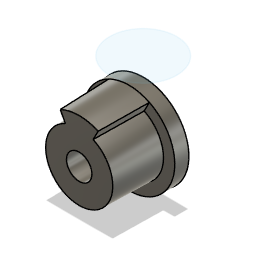
西昊C300头部支撑固定桩 (Autodesk Fusion 360 design; units mm, degrees)
Autodesk Fusion 360 part; units mm, degrees
sketch "草图1" plane through (0, 0, 0) normal (0, 1, 0) x (1, 0, 0)
  circle A0 centre (0, 0) radius 10.35
  dimension "d1" = 20.7
  constraint coincident A0.centre origin
  measures "d1" diameter of A0
extrude "拉伸1" add sketch "草图1" along normal blind 14.5 contours A0 picked at (-1.590097, 1.26806)
sketch "草图2" plane through (0, 14.5, 0) normal (0, 1, 0) x (-1, 0, 0)
  circle A0 centre (0, 0) radius 10.35
  circle A1 centre (0, 0) radius 7.6
  dimension "d4" = 15.2
  constraint coincident A0.centre A1.centre
  measures "d4" diameter of A1
extrude "拉伸2" cut sketch "草图2" against normal blind 11.3 draft -1 contours A0 picked at (9.3948, -0.514196)
sketch "草图3" plane through (0, 14.5, 0) normal (0, 1, 0) x (-1, 0, 0)
  circle A0 centre (0, 0) radius 7.6
  circle A1 centre (0, 0) radius 11.176414
  circle A2 centre (0, 0) radius 9.823441
  constraint coincident A0.centre A1.centre
  constraint concentric A1 A2
extrude "拉伸3" cut sketch "草图3" against normal blind 11.3 contours A1 picked at (10.683813, -0.555253)
sketch "草图6" plane through (0, 3.2, 0) normal (0, 1, 0) x (-1, 0, 0)
  circle A0 centre (0, 0) radius 10.35
  circle A1 centre (0, 0) radius 7.797242
  circle A2 centre (0, 0) radius 10.35
  line L0 (5.18, -3.9) -> (-5.15, -3.9)
  line L1 (-5.15, -3.9) -> (-5.15, -8.97775)
  line L2 (-5.15, -8.97775) -> (5.18, -8.97775)
  line L3 (5.18, -8.97775) -> (5.18, -3.9)
  dimension "d16" = 20.7
  dimension "d18" = 5.15
  dimension "d20" = 10.33
  constraint concentric A0 A2
  constraint horizontal L0
  constraint vertical L1
  constraint horizontal L2
  constraint vertical L3
  measures "d16" diameter of A2
  measures "d18" distance of A0.centre L1
  measures "d20" distance of L1 L3
extrude "拉伸5" add sketch "草图6" along normal blind 11.3 draft -1.5 contours A0 A2 L2 | A0 A1 A2 L1 L2 L3 picked at (1.254031, -9.199184) picked at (0.006674, -8.584239)
sketch "草图7" plane through (0, 14.5, 0) normal (0, 1, 0) x (-1, 0, 0)
  circle A0 centre (0, 0) radius 7.6
sketch "草图8" plane through (0, 14.5, 0) normal (0, 1, 0) x (-1, 0, 0)
sketch "草图9" plane through (0, 14.5, 0) normal (0, 1, 0) x (-1, 0, 0)
sketch "草图10" plane through (0, 14.5, 0) normal (0, 1, 0) x (-1, 0, 0)
  line L0 (-4.854099, -6.475854) -> (-4.854099, -8.804694)
  arc A0 (-4.854099, -8.804694) -> (4.884099, -8.788088) centre (0, 0) ccw
  line L1 (4.884099, -8.788088) -> (4.884099, -6.453258)
  arc A1 (-4.854099, -6.475854) -> (4.884099, -6.453258) centre (0, 0) ccw
  line L2 (4.884099, -6.453258) -> (-4.854099, -6.475854)
  line L3 (0, 0) -> (4.884099, 0)
  line L4 (4.884099, 0) -> (4.884099, -6.453258)
  line L5 (4.884099, -6.453258) -> (0, -6.453258)
  line L6 (0, -6.453258) -> (0, 0)
  line L7 (0, 0) -> (-4.854099, 0)
  line L8 (-4.854099, 0) -> (-4.854099, -6.475854)
  line L9 (-4.854099, -6.475854) -> (0, -6.475854)
  line L10 (0, -6.475854) -> (0, 0)
  constraint horizontal L3
  constraint vertical L4
  constraint horizontal L5
  constraint vertical L6
  constraint coincident A0.centre A1.centre
  constraint horizontal L7
  constraint vertical L8
  constraint horizontal L9
  constraint vertical L10
extrude "拉伸6" add sketch "草图10" against normal blind 11.3 draft 1.5 contours A1 L2 L9 L10 | L2 L6 L7 L8 L10 | L3 L4 L5 L6 L10 picked at (0.012487, -7.540159) picked at (-3.236066, -4.309704) picked at (1.628033, -4.302172)
sketch "草图11" plane through (0, 14.5, 0) normal (0, 1, 0) x (-1, 0, 0)
sketch "草图12" plane through (0, 14.5, 0) normal (0, 1, 0) x (-1, 0, 0)
  line L0 (-4.854099, -6.475854) -> (-4.854099, -8.804694)
  arc A0 (-4.854099, -8.804694) -> (4.884099, -8.788088) centre (0, 0) ccw
  line L1 (4.884099, -8.788088) -> (4.884099, -6.453258)
  line L2 (4.884099, -6.453258) -> (4.011148, -6.455284)
  arc A1 (4.011148, -6.455284) -> (4.014406, -6.453258) centre (0, 0) ccw
  line L3 (4.014406, -6.453258) -> (4.884099, -6.453258)
  line L4 (4.884099, -6.453258) -> (4.884099, -5.822849)
  arc A2 (4.884099, -5.822849) -> (-4.854099, -5.847882) centre (0, 0) ccw
  line L5 (-4.854099, -5.847882) -> (-4.854099, -6.475854)
  line L6 (-4.854099, -6.475854) -> (-3.981148, -6.473829)
  arc A3 (-3.981148, -6.473829) -> (-3.977853, -6.475854) centre (0, 0) ccw
  line L7 (-3.977853, -6.475854) -> (-4.854099, -6.475854)
  line L8 (-4.854099, -5.847882) -> (-4.854099, -8.804694)
  line L9 (4.884099, -8.788088) -> (4.884099, -5.822849)
  line L10 (6.095858, -5.822849) -> (6.095858, -8.804694)
  line L11 (6.095858, -8.804694) -> (4.884099, -8.788088)
  line L12 (6.095858, -5.822849) -> (4.884099, -5.822849)
  line L13 (-4.854099, -8.804694) -> (-6, -8.804694)
  line L14 (-6, -8.804694) -> (-6, -5.822849)
  line L15 (-6, -5.822849) -> (-4.854099, -5.847882)
  constraint parallel L4 L10
  constraint perpendicular L4 L12
  constraint perpendicular L8 L13
  constraint perpendicular L13 L14
extrude "拉伸7" cut sketch "草图12" against normal blind 11.3 draft -1.5 contours L0 L5 L8 L13 L14 L15 | L1 L4 L9 L10 L11 L12 picked at (-5.618033, -7.034466) picked at (5.691938, -7.026934)
sketch "草图13" plane through (0, 0, 0) normal (0, -1, 0) x (1, 0, 0)
  circle A0 centre (0, 0) radius 10.35
  circle A1 centre (0, 0) radius 3.1
  dimension "d28" = 6.2
  constraint concentric A0 A1
  measures "d28" diameter of A1
extrude "拉伸8" cut sketch "草图13" against normal blind 14.5 draft -0.85 contours A1 picked at (-0.459877, 1.40569)
sketch "草图15" plane through (0, 3.2, 0) normal (0, 1, 0) x (-1, 0, 0)
  line L0 (5.18, -5.827914) -> (5.18, -8.960474)
  arc A0 (5.18, -8.960474) -> (-5.15, -8.97775) centre (0, 0) ccw
  line L1 (-5.15, -8.97775) -> (-5.15, -5.854442)
  arc A1 (5.18, -5.827914) -> (-5.15, -5.854442) centre (0, 0) ccw
  line L2 (5.18, -5.827914) -> (-0.020023, -5.827914)
  line L3 (-0.020023, -5.827914) -> (-0.020023, -10.347219)
  line L4 (-0.020023, -10.347219) -> (5.18, -10.347219)
  line L5 (5.18, -10.347219) -> (5.18, -5.827914)
  line L6 (-5.15, -5.854442) -> (-0.020023, -5.854442)
  line L7 (-0.020023, -5.854442) -> (-0.020023, -10.347219)
  line L8 (-0.020023, -10.347219) -> (-5.15, -10.347219)
  line L9 (-5.15, -10.347219) -> (-5.15, -5.854442)
  line L10 (-0.020023, -5.827914) -> (2.779977, -5.827914)
  line L11 (2.779977, -5.827914) -> (2.779977, -10.347219)
  line L12 (2.779977, -10.347219) -> (-0.020023, -10.347219)
  line L13 (-0.020023, -10.347219) -> (-0.020023, -5.827914)
  line L14 (-0.020023, -5.854442) -> (-2.820023, -5.854442)
  line L15 (-2.820023, -5.854442) -> (-2.820023, -10.347219)
  line L16 (-2.820023, -10.347219) -> (-0.020023, -10.347219)
  line L17 (-0.020023, -10.347219) -> (-0.020023, -5.854442)
  circle A2 centre (0, 0) radius 7.797242
  line L18 (5.18, -10.347219) -> (2.779977, -5.827914)
  line L19 (-5.15, -10.347219) -> (-2.820023, -5.854442)
  dimension "d33" = 2.8
  dimension "d34" = 2.8
  constraint horizontal L2
  constraint vertical L3
  constraint horizontal L4
  constraint vertical L5
  constraint horizontal L6
  constraint vertical L7
  constraint horizontal L8
  constraint vertical L9
  constraint horizontal L10
  constraint vertical L11
  constraint horizontal L12
  constraint vertical L13
  constraint horizontal L14
  constraint vertical L15
  constraint horizontal L16
  constraint vertical L17
  constraint concentric A0 A2
extrude "拉伸9" cut sketch "草图15" along normal blind 11.3 draft 1 contours L0 L5 A2 L18 | L1 L9 A2 L19 picked at (4.589689, -8.7734) picked at (-4.572759, -8.777664)
move_body "移动1" bodies 1 to x (1, 0, 0) y (0, 0, 1) z (0, -1, 0) at (0, 0, 0)
sketch "草图14" plane through (0, 14.5, 0) normal (0, 1, 0) x (-1, 0, 0)
  circle A0 centre (0, 0) radius 2.884872
  line L0 (-4.854099, -6.475854) -> (-4.854099, -8.804694)
  arc A1 (-4.854099, -8.804694) -> (4.884099, -8.788088) centre (0, 0) ccw
  line L1 (4.884099, -8.788088) -> (4.884099, -6.453258)
  line L2 (4.884099, -6.453258) -> (4.011148, -6.455284)
  arc A2 (4.011148, -6.455284) -> (4.014406, -6.453258) centre (0, 0) ccw
  line L3 (4.014406, -6.453258) -> (4.884099, -6.453258)
  line L4 (4.884099, -6.453258) -> (4.884099, -5.822849)
  arc A3 (4.884099, -5.822849) -> (-4.854099, -5.847882) centre (0, 0) ccw
  line L5 (-4.854099, -5.847882) -> (-4.854099, -6.475854)
  line L6 (-4.854099, -6.475854) -> (-3.981148, -6.473829)
  arc A4 (-3.981148, -6.473829) -> (-3.977853, -6.475854) centre (0, 0) ccw
  line L7 (-3.977853, -6.475854) -> (-4.854099, -6.475854)
  line L8 (-4.854099, -5.847882) -> (0.017145, -5.847882)
  line L9 (0.017145, -5.847882) -> (0.017145, -10.054084)
  line L10 (0.017145, -10.054084) -> (-4.854099, -10.054084)
  line L11 (-4.854099, -10.054084) -> (-4.854099, -5.847882)
  line L12 (4.884099, -5.822849) -> (0.017145, -5.822849)
  line L13 (0.017145, -5.822849) -> (0.017145, -10.054084)
  line L14 (0.017145, -10.054084) -> (4.884099, -10.054084)
  line L15 (4.884099, -10.054084) -> (4.884099, -5.822849)
  line L16 (0.017145, -10.054084) -> (2.817145, -10.054084)
  line L17 (2.817145, -10.054084) -> (2.817145, -5.822849)
  line L18 (2.817145, -5.822849) -> (0.017145, -5.822849)
  line L19 (0.017145, -5.822849) -> (0.017145, -10.054084)
  line L20 (0.017145, -10.054084) -> (-2.782855, -10.054084)
  line L21 (-2.782855, -10.054084) -> (-2.782855, -5.847882)
  line L22 (-2.782855, -5.847882) -> (0.017145, -5.847882)
  line L23 (0.017145, -5.847882) -> (0.017145, -10.054084)
  circle A5 centre (0, 0) radius 7.6
  line L24 (4.884099, -8.788088) -> (2.817145, -5.822849)
  line L25 (-4.854099, -8.804694) -> (-2.782855, -5.847882)
  dimension "d31" = 2.8
  dimension "d32" = 2.8
  constraint horizontal L8
  constraint vertical L9
  constraint horizontal L10
  constraint vertical L11
  constraint horizontal L12
  constraint vertical L13
  constraint horizontal L14
  constraint vertical L15
  constraint horizontal L16
  constraint vertical L17
  constraint horizontal L18
  constraint vertical L19
  constraint horizontal L20
  constraint vertical L21
  constraint horizontal L22
  constraint vertical L23
  constraint concentric A0 A5
sketch "草图4" plane through (0, 14.5, 0) normal (0, 1, 0) x (-1, 0, 0)
  circle A0 centre (0, 0) radius 7.6
  line L0 (7.6, -10.35) -> (-7.6, -10.35)
  line L1 (-7.6, -10.35) -> (-7.6, -7.6)
  line L2 (-7.6, -7.6) -> (7.6, -7.6)
  line L3 (7.6, -7.6) -> (7.6, -10.35)
  circle A1 centre (0, -10.35) radius 7.6
  circle A2 centre (0, 0) radius 10.35
  circle A3 centre (0, 0) radius 12.840658
  dimension "d9" = 7.6
  dimension "d10" = 7.6
  dimension "d11" = 15.2
  dimension "d12" = 10.35
  dimension "d15" = 20.7
  constraint horizontal L0
  constraint vertical L1
  constraint horizontal L2
  constraint vertical L3
  constraint midpoint L0 A1.centre
  constraint coincident L0.end A1
  constraint concentric A0 A2
  constraint concentric A0 A3
  constraint coincident L0.end A3
  measures "d9" distance of A0.centre L2
  measures "d10" distance of A0.centre L1
  measures "d11" distance of L1 L3
  measures "d12" distance of A0.centre L0
  measures "d15" diameter of A2
extrude "拉伸4" [rolled back] along distance -11.3 taper angle 0
sketch "草图5" plane through (0, 14.5, 0) normal (0, 1, 0) x (-1, 0, 0)
  arc A0 (5.565912, -5.175) -> (-5.565912, -5.175) centre (0, 0) ccw
  arc A1 (-5.565912, -5.175) -> (-7.6, -10.35) centre (0, -10.35) ccw
  line L0 (-7.6, -10.35) -> (7.6, -10.35)
  arc A2 (7.6, -10.35) -> (5.565912, -5.175) centre (0, -10.35) ccw
